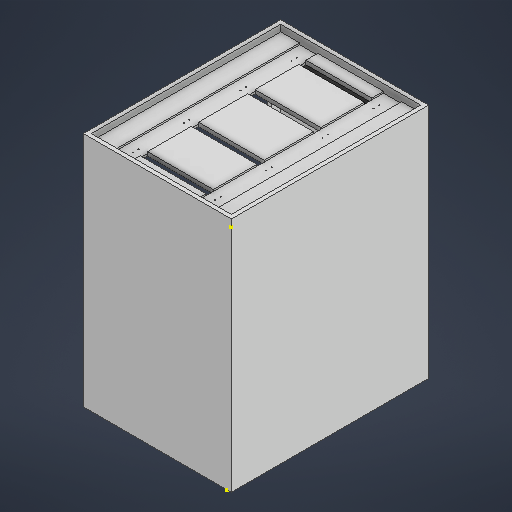
# Autodesk Inventor part: box
Saved by Autodesk Inventor 2027.1 (Build 311270010, 270A)
## iProperties
Created: 2026-10-02
Part Number: box
Material: Generic
Document SubType Name: Modeling
Designer: Arik
Density: 1 g/cm^3
Appearance: Default
Author: Arik
Autodesk Inventor part; units mm, degrees
ref_plane "YZ Plane" through (0, 0, 0) normal (1, 0, 0) x (0, 1, 0)
ref_plane "XZ Plane" through (0, 0, 0) normal (0, 1, 0) x (-1, 0, 0)
ref_plane "XY Plane" through (0, 0, 0) normal (0, 0, 1) x (1, 0, 0)
sketch "Sketch1" plane through (0, 0, 0) normal (0, 1, 0) x (-1, 0, 0)
  line L0 (0, 0) -> (450, 0)
  line L1 (450, 0) -> (450, -600)
  line L2 (450, -600) -> (0, -600)
  line L3 (0, -600) -> (0, 0)
  dimension "d0" = 450
  dimension "d1" = 600
  constraints: 8 end point, 2 parallel, 1 horizontal, 1 perpendicular
  measures "d0" distance of L1.end L2.end
  measures "d1" distance of L0.end L1.end
extrude "Extrusion1" add sketch "Sketch1" along normal blind 12
sketch "Sketch2" plane through (0, 12, 0) normal (0, 1, 0) x (1, 0, 0)
  line L0 (0, 0) -> (0, 600) projected
  line L1 (-450, 600) -> (-450, 0) projected
  line L2 (0, 600) -> (-450, 600)
  line L3 (-450, 600) -> (-450, 0)
  line L4 (-450, 0) -> (0, 0)
  line L5 (0, 0) -> (0, 600)
  line L6 (-438, 588) -> (-12, 588)
  line L7 (-12, 588) -> (-12, 12)
  line L8 (-12, 12) -> (-438, 12)
  line L9 (-438, 12) -> (-438, 588)
  dimension "d4" = 12
  constraints: 16 end point, 4 parallel, 2 perpendicular, 1 horizontal, 3 other
  measures "d4" distance between parallel lines of L2 L6
extrude "Extrusion2" add sketch "Sketch2" along normal blind 708
sketch "Sketch3" plane through (-450, 0, -600) normal (-1, 0, 0) x (0, 0, 1)
  line L0 (0, 0) -> (40, 0)
  line L1 (40, 0) -> (40, 100)
  line L2 (40, 100) -> (0, 100)
  line L3 (0, 100) -> (0, 0)
  line L4 (600, 0) -> (560, 0)
  line L5 (560, 0) -> (560, 100)
  line L6 (560, 100) -> (600, 100)
  line L7 (600, 100) -> (600, 0)
  line L8 (600, 720) -> (560, 720)
  line L9 (560, 720) -> (560, 620)
  line L10 (560, 620) -> (600, 620)
  line L11 (600, 620) -> (600, 720)
  line L12 (40, 100) -> (560, 100)
  line L13 (560, 100) -> (560, 620)
  line L14 (560, 620) -> (40, 620)
  line L15 (40, 620) -> (40, 100)
  dimension "d7" = 40
  dimension "d8" = 100
  dimension "d9" = 40
  dimension "d10" = 100
  dimension "d11" = 40
  dimension "d12" = 100
  constraints: 32 end point, 8 parallel, 4 horizontal, 4 perpendicular, 1 point on line
  measures "d7" distance of L2.end L1.end
  measures "d8" distance of L1.end L0.end
  measures "d9" distance of L5.end L6.end
  measures "d10" distance of L4.end L5.end
  measures "d11" distance of L10.end L9.end
  measures "d12" distance of L9.end L8.end
extrude "Extrusion3" cut sketch "Sketch3" against normal blind 12 contours L15 L14 L13 L12
sketch "Sketch4" plane through (-12, 12, -588) normal (-1, 0, 0) x (0, 0, 1)
  point P0 (588, -12)
sketch "Sketch5" plane through (-12, 12, -588) normal (-1, 0, 0) x (0, 0, 1)
  line L0 (0, 0) -> (0, 708) projected
  line L1 (0, 708) -> (0, 688)
  line L2 (576, 0) -> (576, 708) projected
  line L3 (0, 688) -> (576, 688)
  line L4 (576, 688) -> (576, 676)
  line L5 (576, 676) -> (0, 676)
  line L6 (0, 676) -> (0, 688)
  point P0 (588, -12)
  dimension "d15" = 20
  dimension "d16" = 12
  constraints: 10 end point, 2 parallel, 2 point on line, 1 horizontal, 1 perpendicular
  measures "d15" distance of L0.end L1.end
  measures "d16" distance of L3.end L4.end
extrude "Extrusion4" add sketch "Sketch5" along normal up to surface (438 mm away)
sketch "Sketch6" plane through (-12, 700, -12) normal (0, 1, 0) x (1, 0, 0)
  line L0 (-426, 576) -> (0, 576) projected
  line L1 (-213, 576) -> (-213, 0)
  line L2 (0, 0) -> (-426, 0) projected
  line L3 (-213, 576) -> (-213, 504)
  line L4 (-213, 504) -> (-213, 515)
  line L5 (-213, 515) -> (-113, 515)
  line L6 (-213, 540) -> (-113, 540)
  line L7 (-113, 540) -> (-313, 540)
  line L8 (-313, 540) -> (-313, 518)
  line L9 (-313, 518) -> (-113, 518)
  line L10 (-113, 518) -> (-113, 540)
  line L11 (-213, 529) -> (-338, 529)
  line L12 (-338, 529) -> (-338, 537.5)
  circle A0 centre (-338, 537.5) radius 1.5
  line L13 (-338, 537.5) -> (-338, 520.5)
  circle A1 centre (-338, 520.5) radius 1.5
  circle A2 centre (-88, 537.5) radius 1.5
  circle A3 centre (-88, 520.5) radius 1.5
  line L14 (-213, 518) -> (-213, 374)
  line L15 (-213, 374) -> (-213, 385)
  line L16 (-213, 385) -> (-113, 385)
  line L17 (-113, 385) -> (-313, 385)
  line L18 (-313, 385) -> (-313, 363)
  line L19 (-313, 363) -> (-113, 363)
  line L20 (-113, 363) -> (-113, 385)
  line L21 (-88, 537.5) -> (-88, 520.5)
  line L22 (-113, 374) -> (-88, 374)
  line L23 (-88, 374) -> (-88, 382.5)
  line L24 (-88, 382.5) -> (-88, 365.5)
  circle A4 centre (-88, 382.5) radius 1.5
  circle A5 centre (-88, 365.5) radius 1.5
  circle A6 centre (-338, 382.5) radius 1.5
  circle A7 centre (-338, 365.5) radius 1.5
  line L25 (-213, 288) -> (-149.1067, 288)
  line L26 (-113, 36) -> (-313, 36)
  line L27 (-313, 36) -> (-313, 58)
  line L28 (-313, 58) -> (-113, 58)
  line L29 (-113, 58) -> (-113, 36)
  circle A8 centre (-338, 38.5) radius 1.5
  circle A9 centre (-338, 55.5) radius 1.5
  circle A10 centre (-88, 38.5) radius 1.5
  circle A11 centre (-88, 55.5) radius 1.5
  line L30 (-213, 191) -> (-113, 191)
  line L31 (-113, 191) -> (-313, 191)
  line L32 (-313, 191) -> (-313, 213)
  line L33 (-313, 213) -> (-113, 213)
  line L34 (-113, 213) -> (-113, 191)
  circle A12 centre (-88, 193.5) radius 1.5
  circle A13 centre (-88, 210.5) radius 1.5
  circle A14 centre (-338, 193.5) radius 1.5
  circle A15 centre (-338, 210.5) radius 1.5
  point P0 (12, -12)
  point P1 (-113, 202)
  dimension "d19" = 72
  dimension "d20" = 11
  dimension "d21" = 100
  dimension "d22" = 200
  dimension "d23" = 22
  dimension "d24" = 125
  dimension "d25" = 8.5
  dimension "d26" = 3
  dimension "d27" = 17
  dimension "d28" = 3
  dimension "d29" = 144
  dimension "d30" = 11
  dimension "d31" = 100
  dimension "d32" = 22
  dimension "d33" = 25
  dimension "d34" = 8.5
  dimension "d35" = 17
  constraints: 66 end point, 22 symmetric about line, 16 centre point, 6 midpoint, 6 perpendicular, 6 point on line, 5 horizontal, 4 coincident, 4 parallel, 3 vertical, 12 other
  measures "d19" distance of L1.start L3.end
  measures "d20" distance of L3.end L4.end
  measures "d21" distance of L4.end L5.end
  measures "d22" distance of L9.end L8.end
  measures "d23" distance of L8.end L7.end
  measures "d24" distance of L11.start L11.end
  measures "d25" distance of L11.end L12.end
  measures "d26" diameter of A0
  measures "d27" distance of L13.start L13.end
  measures "d28" diameter of A1
  measures "d29" distance of L14.start L14.end
  measures "d30" distance of L14.end L15.end
  measures "d31" distance of L15.end L16.end
  measures "d32" distance of L18.end L17.end
  measures "d33" distance of L22.start L22.end
  measures "d34" distance of L22.end L23.end
  measures "d35" distance of L23.end L24.end
extrude "Extrusion5" cut sketch "Sketch6" against normal blind 12
sketch "Sketch7" plane through (-12, 700, -12) normal (0, 1, 0) x (1, 0, 0)
  point P0 (12, -12)
sketch "Sketch8" plane through (-12, 700, -12) normal (0, 1, 0) x (1, 0, 0)
  line L0 (-313, 36) -> (-113, 36) projected
  line L1 (0, 0) -> (-426, 0) projected
  line L2 (-113, 36) -> (-58, 36)
  line L3 (-58, 36) -> (-58, 0)
  line L4 (-58, 0) -> (-113, 0)
  line L5 (-113, 0) -> (-113, 36)
  line L6 (0, 576) -> (-426, 576) projected
  line L7 (-58, 0) -> (-113, 0)
  line L8 (-113, 0) -> (-113, 576)
  line L9 (-113, 576) -> (-58, 576)
  line L10 (-58, 576) -> (-58, 0)
  line L11 (-213, 576) -> (-213, 492.9695)
  line L12 (-426, 0) -> (0, 0)
  line L13 (-368, 0) -> (-313, 0)
  line L14 (-426, 576) -> (0, 576)
  line L15 (-313, 0) -> (-313, 576)
  line L16 (-313, 576) -> (-368, 576)
  line L17 (-368, 576) -> (-368, 0)
  line L18 (-313, 518) -> (-113, 518) projected
  line L19 (-313, 540) -> (-113, 540) projected
  line L20 (-313, 518) -> (-313, 540)
  point P0 (12, -12)
  dimension "d38" = 55
  constraints: 32 end point, 9 symmetric about line, 5 point on line, 4 parallel, 2 horizontal, 2 perpendicular, 2 vertical, 1 midpoint
  measures "d38" distance of L3.end L4.end
extrude "Extrusion6" cut sketch "Sketch8" against normal blind 5 contours L15 L1 L17 L6 | L8 L6 L10 L2 | L2 L3 L1 L5
body "Solid1"
